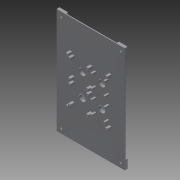
# Autodesk Inventor part: SimpleLensPlane
Saved by Autodesk Inventor 2015 (Build 190159000, 159)
## iProperties
Created: 2015-03-20
Part Number: SimpleLensPlane
Material: NylonD2W
Document SubType Name: Modeling
Designer: Akovo_000
Density: 0.93 g/cm^3
Appearance: Nylon 6
Mass: 35.1863 g
Surface Area: 486.293 cm^2
Volume: 37.8348 cm^3
Author: Akovo_000
Autodesk Inventor part; units mm, degrees
ref_plane "YZ Plane" through (0, 0, 0) normal (1, 0, 0) x (0, 1, 0)
ref_plane "XZ Plane" through (0, 0, 0) normal (0, 1, 0) x (-1, 0, 0)
ref_plane "Main Work Pane" through (0, 2.75, 7) normal (0, 1, 0) x (-1, 0, 0)
sketch "Panel" plane through (0, 2.75, 7) normal (0, 1, 0) x (-1, 0, 0)
  circle A0 centre (9.841, 27.1334) radius 5.8
  circle A1 centre (9.841, -11.8666) radius 5.8
  circle A2 centre (43.641, -11.8666) radius 5.8
  circle A3 centre (43.641, 27.1334) radius 5.8
  line L0 (61.641, 45.1334) -> (25.641, 45.1334)
  line L1 (25.641, 45.1334) -> (25.641, 9.1334)
  line L2 (25.641, 9.1334) -> (61.641, 9.1334)
  line L3 (61.641, 9.1334) -> (61.641, 45.1334)
  line L4 (61.641, 45.1334) -> (25.641, 9.1334) construction
  line L5 (25.641, 45.1334) -> (61.641, 9.1334) construction
  line L6 (61.641, 6.1334) -> (25.641, 6.1334)
  line L7 (25.641, 6.1334) -> (25.641, -29.8666)
  line L8 (25.641, -29.8666) -> (61.641, -29.8666)
  line L9 (61.641, -29.8666) -> (61.641, 6.1334)
  line L10 (61.641, 6.1334) -> (25.641, -29.8666) construction
  line L11 (25.641, 6.1334) -> (61.641, -29.8666) construction
  line L12 (22.641, 39.9334) -> (-2.959, 39.9334)
  line L13 (-2.959, 39.9334) -> (-2.959, 14.3334)
  line L14 (-2.959, 14.3334) -> (22.641, 14.3334)
  line L15 (22.641, 14.3334) -> (22.641, 39.9334)
  line L16 (22.641, 39.9334) -> (-2.959, 14.3334) construction
  line L17 (-2.959, 39.9334) -> (22.641, 14.3334) construction
  line L18 (22.641, 0.9334) -> (-2.959, 0.9334)
  line L19 (-2.959, 0.9334) -> (-2.959, -24.6666)
  line L20 (-2.959, -24.6666) -> (22.641, -24.6666)
  line L21 (22.641, -24.6666) -> (22.641, 0.9334)
  line L22 (22.641, 0.9334) -> (-2.959, -24.6666) construction
  line L23 (-2.959, 0.9334) -> (22.641, -24.6666) construction
  line L24 (61.641, -29.8666) -> (61.641, 45.1334)
  line L25 (61.641, 45.1334) -> (-2.959, 45.1334)
  line L26 (-2.959, 45.1334) -> (-2.959, -29.8666)
  line L27 (-2.959, -29.8666) -> (61.641, -29.8666)
  line L28 (88.341, -83.8666) -> (-29.659, -83.8666)
  line L29 (-29.659, -83.8666) -> (-29.659, 99.1334)
  line L30 (-29.659, 99.1334) -> (88.341, 99.1334)
  line L31 (88.341, 99.1334) -> (88.341, -83.8666)
  line L32 (43.641, 21.3334) -> (43.641, -6.0666) construction
  line L33 (37.841, 27.1334) -> (15.641, 27.1334) construction
  line L34 (9.841, 21.3334) -> (9.841, -6.0666) construction
  line L35 (15.641, -11.8666) -> (37.841, -11.8666) construction
  line L36 (17.4252, 99.1334) -> (17.4252, 45.1334) construction
  line L37 (17.4252, -29.8666) -> (17.4252, -83.8666) construction
  line L38 (61.641, 7.6334) -> (88.341, 7.6334) construction
  line L39 (-2.959, 7.6334) -> (-29.659, 7.6334) construction
  circle A4 centre (80.841, 91.1334) radius 2
  circle A5 centre (-22.159, 91.1334) radius 2
  circle A6 centre (80.841, -75.8666) radius 2
  circle A7 centre (-22.159, -75.8666) radius 2
  line L40 (67.962, 75.8227) -> (67.962, -63.4589)
  line L41 (67.962, -63.4589) -> (-9.8153, -63.4589)
  line L42 (-9.8153, -63.4589) -> (-9.8153, 75.8227)
  line L43 (-9.8153, 75.8227) -> (67.962, 75.8227)
  line L44 (-22.159, 99.1334) -> (-22.159, 91.1334) construction
  line L45 (-22.159, 91.1334) -> (-29.659, 91.1334) construction
  line L46 (80.841, 99.1334) -> (80.841, 91.1334) construction
  line L47 (80.841, 91.1334) -> (88.341, 91.1334) construction
  line L48 (88.341, -75.8666) -> (80.841, -75.8666) construction
  line L49 (80.841, -75.8666) -> (80.841, -83.8666) construction
  line L50 (-22.159, -83.8666) -> (-22.159, -75.8666) construction
  line L51 (-22.159, -75.8666) -> (-29.659, -75.8666) construction
  dimension "d337" = 11.6
  dimension "d490" = 36
  dimension "d491" = 36
  dimension "d494" = 3
  dimension "d495" = 25.6
  dimension "d496" = 25.6
  dimension "d497" = 3
  dimension "d498" = 0
  dimension "d593" = 4
  dimension "d674" = 183
  dimension "d675" = 118
  dimension "d676" = 7.5
  dimension "d677" = 8
  constraints: 104 end point, 20 perpendicular, 14 equal length, 12 midpoint, 12 parallel, 12 point on line, 8 centre point, 8 point on circle, 6 equal radius, 6 line through centre, 5 horizontal, 3 vertical, 2 collinear, 3 other
  measures "d337" diameter of A2
  measures "d490" distance of L2.end L1.end
  measures "d491" distance of L1.end L0.end
  measures "d494" distance between parallel lines of L6 L2
  measures "d495" distance of L14.end L13.end
  measures "d496" distance of L13.end L12.end
  measures "d497" distance between parallel lines of L21 L7
  measures "d498" distance between parallel lines of L26 L13
  measures "d593" diameter of A4
  measures "d674" distance between parallel lines of L28 L30
  measures "d675" distance between parallel lines of L29 L31
  measures "d676" distance of L44.end L45.end
  measures "d677" distance of L44.start L44.end
extrude "FlatPlane" add sketch "Panel" along normal blind 1.5 contours L3 L2 L1 L0 | L1 L2 L24 L6 L7 L27 L26 L20 L21 L18 L14 L15 L12 L25 | L9 L8 L7 L6 | L12 L15 L14 L13 | L18 L21 L20 L19 | L28 L29 L30 L31 | L40 L41 L42 L43
sketch "BoardSuport" plane through (0, 2.75, 7) normal (0, -1, 0) x (1, 0, 0)
  line L0 (-59.141, 42.6334) -> (-28.141, 42.6334) construction
  line L1 (-28.141, 42.6334) -> (-28.141, 11.6334) construction
  line L2 (-28.141, 11.6334) -> (-59.141, 11.6334) construction
  line L3 (-59.141, 11.6334) -> (-59.141, 42.6334) construction
  circle A0 centre (-43.641, 27.1334) radius 5.8
  line L4 (-59.141, 42.6334) -> (-28.141, 11.6334) construction
  line L5 (-28.141, 42.6334) -> (-59.141, 11.6334) construction
  line L6 (-59.141, 3.6334) -> (-28.141, 3.6334) construction
  line L7 (-28.141, 3.6334) -> (-28.141, -27.3666) construction
  line L8 (-28.141, -27.3666) -> (-59.141, -27.3666) construction
  line L9 (-59.141, -27.3666) -> (-59.141, 3.6334) construction
  circle A1 centre (-43.641, -11.8666) radius 5.8
  line L10 (-59.141, 3.6334) -> (-28.141, -27.3666) construction
  line L11 (-28.141, 3.6334) -> (-59.141, -27.3666) construction
  line L12 (-21.091, 38.3834) -> (1.409, 38.3834) construction
  line L13 (1.409, 38.3834) -> (1.409, 15.8834) construction
  line L14 (1.409, 15.8834) -> (-21.091, 15.8834) construction
  line L15 (-21.091, 15.8834) -> (-21.091, 38.3834) construction
  circle A2 centre (-9.841, 27.1334) radius 5.8
  line L16 (-21.091, 38.3834) -> (1.409, 15.8834) construction
  line L17 (1.409, 38.3834) -> (-21.091, 15.8834) construction
  line L18 (-21.091, -0.6166) -> (1.409, -0.6166) construction
  line L19 (1.409, -0.6166) -> (1.409, -23.1166) construction
  line L20 (1.409, -23.1166) -> (-21.091, -23.1166) construction
  line L21 (-21.091, -23.1166) -> (-21.091, -0.6166) construction
  circle A3 centre (-9.841, -11.8666) radius 5.8
  line L22 (-21.091, -0.6166) -> (1.409, -23.1166) construction
  line L23 (1.409, -0.6166) -> (-21.091, -23.1166) construction
  line L24 (-61.241, 5.7334) -> (-57.041, 5.7334)
  line L25 (-57.041, 5.7334) -> (-57.041, 1.5334)
  line L26 (-57.041, 1.5334) -> (-61.241, 1.5334)
  line L27 (-61.241, 1.5334) -> (-61.241, 5.7334)
  line L28 (-61.241, 5.7334) -> (-57.041, 1.5334) construction
  line L29 (-57.041, 5.7334) -> (-61.241, 1.5334) construction
  line L30 (-61.241, 13.7334) -> (-57.041, 13.7334)
  line L31 (-57.041, 13.7334) -> (-57.041, 9.5334)
  line L32 (-57.041, 9.5334) -> (-61.241, 9.5334)
  line L33 (-61.241, 9.5334) -> (-61.241, 13.7334)
  line L34 (-61.241, 13.7334) -> (-57.041, 9.5334) construction
  line L35 (-57.041, 13.7334) -> (-61.241, 9.5334) construction
  line L36 (-30.241, 13.7334) -> (-26.041, 13.7334)
  line L37 (-26.041, 13.7334) -> (-26.041, 9.5334)
  line L38 (-26.041, 9.5334) -> (-30.241, 9.5334)
  line L39 (-30.241, 9.5334) -> (-30.241, 13.7334)
  line L40 (-30.241, 13.7334) -> (-26.041, 9.5334) construction
  line L41 (-26.041, 13.7334) -> (-30.241, 9.5334) construction
  line L42 (-30.241, 44.7334) -> (-26.041, 44.7334)
  line L43 (-26.041, 44.7334) -> (-26.041, 40.5334)
  line L44 (-26.041, 40.5334) -> (-30.241, 40.5334)
  line L45 (-30.241, 40.5334) -> (-30.241, 44.7334)
  line L46 (-30.241, 44.7334) -> (-26.041, 40.5334) construction
  line L47 (-26.041, 44.7334) -> (-30.241, 40.5334) construction
  line L48 (-61.241, 44.7334) -> (-57.041, 44.7334)
  line L49 (-57.041, 44.7334) -> (-57.041, 40.5334)
  line L50 (-57.041, 40.5334) -> (-61.241, 40.5334)
  line L51 (-61.241, 40.5334) -> (-61.241, 44.7334)
  line L52 (-61.241, 44.7334) -> (-57.041, 40.5334) construction
  line L53 (-57.041, 44.7334) -> (-61.241, 40.5334) construction
  line L54 (-30.241, 5.7334) -> (-26.041, 5.7334)
  line L55 (-26.041, 5.7334) -> (-26.041, 1.5334)
  line L56 (-26.041, 1.5334) -> (-30.241, 1.5334)
  line L57 (-30.241, 1.5334) -> (-30.241, 5.7334)
  line L58 (-30.241, 5.7334) -> (-26.041, 1.5334) construction
  line L59 (-26.041, 5.7334) -> (-30.241, 1.5334) construction
  line L60 (-30.241, -25.2666) -> (-26.041, -25.2666)
  line L61 (-26.041, -25.2666) -> (-26.041, -29.4666)
  line L62 (-26.041, -29.4666) -> (-30.241, -29.4666)
  line L63 (-30.241, -29.4666) -> (-30.241, -25.2666)
  line L64 (-30.241, -25.2666) -> (-26.041, -29.4666) construction
  line L65 (-26.041, -25.2666) -> (-30.241, -29.4666) construction
  line L66 (-61.241, -25.2666) -> (-57.041, -25.2666)
  line L67 (-57.041, -25.2666) -> (-57.041, -29.4666)
  line L68 (-57.041, -29.4666) -> (-61.241, -29.4666)
  line L69 (-61.241, -29.4666) -> (-61.241, -25.2666)
  line L70 (-61.241, -25.2666) -> (-57.041, -29.4666) construction
  line L71 (-57.041, -25.2666) -> (-61.241, -29.4666) construction
  line L72 (-22.591, -21.6166) -> (-19.591, -21.6166)
  line L73 (-19.591, -21.6166) -> (-19.591, -24.6166)
  line L74 (-19.591, -24.6166) -> (-22.591, -24.6166)
  line L75 (-22.591, -24.6166) -> (-22.591, -21.6166)
  line L76 (-22.591, -21.6166) -> (-19.591, -24.6166) construction
  line L77 (-19.591, -21.6166) -> (-22.591, -24.6166) construction
  line L78 (-0.091, -21.6166) -> (2.909, -21.6166)
  line L79 (2.909, -21.6166) -> (2.909, -24.6166)
  line L80 (2.909, -24.6166) -> (-0.091, -24.6166)
  line L81 (-0.091, -24.6166) -> (-0.091, -21.6166)
  line L82 (-0.091, -21.6166) -> (2.909, -24.6166) construction
  line L83 (2.909, -21.6166) -> (-0.091, -24.6166) construction
  line L84 (-0.091, 0.8834) -> (2.909, 0.8834)
  line L85 (2.909, 0.8834) -> (2.909, -2.1166)
  line L86 (2.909, -2.1166) -> (-0.091, -2.1166)
  line L87 (-0.091, -2.1166) -> (-0.091, 0.8834)
  line L88 (-0.091, 0.8834) -> (2.909, -2.1166) construction
  line L89 (2.909, 0.8834) -> (-0.091, -2.1166) construction
  line L90 (-22.591, 0.8834) -> (-19.591, 0.8834)
  line L91 (-19.591, 0.8834) -> (-19.591, -2.1166)
  line L92 (-19.591, -2.1166) -> (-22.591, -2.1166)
  line L93 (-22.591, -2.1166) -> (-22.591, 0.8834)
  line L94 (-22.591, 0.8834) -> (-19.591, -2.1166) construction
  line L95 (-19.591, 0.8834) -> (-22.591, -2.1166) construction
  line L96 (-22.591, 14.3834) -> (-19.591, 14.3834)
  line L97 (-19.591, 14.3834) -> (-19.591, 17.3834)
  line L98 (-19.591, 17.3834) -> (-22.591, 17.3834)
  line L99 (-22.591, 17.3834) -> (-22.591, 14.3834)
  line L100 (-22.591, 14.3834) -> (-19.591, 17.3834) construction
  line L101 (-19.591, 14.3834) -> (-22.591, 17.3834) construction
  line L102 (2.909, 14.3834) -> (-0.091, 14.3834)
  line L103 (-0.091, 14.3834) -> (-0.091, 17.3834)
  line L104 (-0.091, 17.3834) -> (2.909, 17.3834)
  line L105 (2.909, 17.3834) -> (2.909, 14.3834)
  line L106 (2.909, 14.3834) -> (-0.091, 17.3834) construction
  line L107 (-0.091, 14.3834) -> (2.909, 17.3834) construction
  line L108 (2.909, 39.8834) -> (-0.091, 39.8834)
  line L109 (-0.091, 39.8834) -> (-0.091, 36.8834)
  line L110 (-0.091, 36.8834) -> (2.909, 36.8834)
  line L111 (2.909, 36.8834) -> (2.909, 39.8834)
  line L112 (2.909, 39.8834) -> (-0.091, 36.8834) construction
  line L113 (-0.091, 39.8834) -> (2.909, 36.8834) construction
  line L114 (-22.591, 39.8834) -> (-19.591, 39.8834)
  line L115 (-19.591, 39.8834) -> (-19.591, 36.8834)
  line L116 (-19.591, 36.8834) -> (-22.591, 36.8834)
  line L117 (-22.591, 36.8834) -> (-22.591, 39.8834)
  line L118 (-22.591, 39.8834) -> (-19.591, 36.8834) construction
  line L119 (-19.591, 39.8834) -> (-22.591, 36.8834) construction
  arc A4 (-59.141, 40.5334) -> (-57.041, 42.6334) centre (-59.141, 42.6334) ccw
  arc A5 (-30.241, 42.6334) -> (-28.141, 40.5334) centre (-28.141, 42.6334) ccw
  arc A6 (-28.141, 13.7334) -> (-30.241, 11.6334) centre (-28.141, 11.6334) ccw
  arc A7 (-57.041, 11.6334) -> (-59.141, 13.7334) centre (-59.141, 11.6334) ccw
  arc A8 (-59.141, 1.5334) -> (-57.041, 3.6334) centre (-59.141, 3.6334) ccw
  arc A9 (-57.041, -27.3666) -> (-59.141, -25.2666) centre (-59.141, -27.3666) ccw
  arc A10 (-28.141, -25.2666) -> (-30.241, -27.3666) centre (-28.141, -27.3666) ccw
  arc A11 (-19.591, -23.1166) -> (-21.091, -21.6166) centre (-21.091, -23.1166) ccw
  arc A12 (1.409, -21.6166) -> (-0.091, -23.1166) centre (1.409, -23.1166) ccw
  arc A13 (-0.091, -0.6166) -> (1.409, -2.1166) centre (1.409, -0.6166) ccw
  arc A14 (-21.091, -2.1166) -> (-19.591, -0.6166) centre (-21.091, -0.6166) ccw
  arc A15 (-30.241, 3.6334) -> (-28.141, 1.5334) centre (-28.141, 3.6334) ccw
  arc A16 (-21.091, 36.8834) -> (-19.591, 38.3834) centre (-21.091, 38.3834) ccw
  arc A17 (-19.591, 15.8834) -> (-21.091, 17.3834) centre (-21.091, 15.8834) ccw
  arc A18 (1.409, 17.3834) -> (-0.091, 15.8834) centre (1.409, 15.8834) ccw
  arc A19 (-0.091, 38.3834) -> (1.409, 36.8834) centre (1.409, 38.3834) ccw
  circle A20 centre (-59.141, 42.6334) radius 0.9
  circle A21 centre (-59.141, 11.6334) radius 0.9
  circle A22 centre (-28.141, 11.6334) radius 0.9
  circle A23 centre (-28.141, 42.6334) radius 0.9
  circle A24 centre (-59.141, 3.6334) radius 0.9
  circle A25 centre (-59.141, -27.3666) radius 0.9
  circle A26 centre (-28.141, -27.3666) radius 0.9
  circle A27 centre (-28.141, 3.6334) radius 0.9
  circle A28 centre (-21.091, -0.6166) radius 0.9
  circle A29 centre (-21.091, -23.1166) radius 0.9
  circle A30 centre (1.409, -23.1166) radius 0.9
  circle A31 centre (1.409, -0.6166) radius 0.9
  circle A32 centre (1.409, 15.8834) radius 0.9
  circle A33 centre (-21.091, 15.8834) radius 0.9
  circle A34 centre (1.409, 38.3834) radius 0.9
  circle A35 centre (-21.091, 38.3834) radius 0.9
  circle A36 centre (-43.641, 27.1334) radius 5.8 projected
  circle A37 centre (-9.841, 27.1334) radius 5.8 projected
  circle A38 centre (-43.641, -11.8666) radius 5.8 projected
  circle A39 centre (-9.841, -11.8666) radius 5.8 projected
  line L120 (-61.241, 44.7334) -> (2.909, 44.7334) construction
  line L121 (2.909, 44.7334) -> (2.909, -29.4666) construction
  line L122 (2.909, -29.4666) -> (-61.241, -29.4666) construction
  line L123 (-61.241, -29.4666) -> (-61.241, 44.7334) construction
  line L124 (-61.241, 44.7334) -> (-65.241, 44.7334)
  line L125 (-65.241, 44.7334) -> (-65.241, 48.7334)
  line L126 (-65.241, 48.7334) -> (-61.241, 48.7334)
  line L127 (-61.241, 48.7334) -> (-61.241, 44.7334)
  line L128 (-61.241, -29.4666) -> (-65.241, -29.4666)
  line L129 (-65.241, -29.4666) -> (-65.241, -33.4666)
  line L130 (-65.241, -33.4666) -> (-61.241, -33.4666)
  line L131 (-61.241, -33.4666) -> (-61.241, -29.4666)
  line L132 (2.909, -29.4666) -> (6.909, -29.4666)
  line L133 (6.909, -29.4666) -> (6.909, -33.4666)
  line L134 (6.909, -33.4666) -> (2.909, -33.4666)
  line L135 (2.909, -33.4666) -> (2.909, -29.4666)
  line L136 (2.909, 44.7334) -> (6.909, 44.7334)
  line L137 (6.909, 44.7334) -> (6.909, 48.7334)
  line L138 (6.909, 48.7334) -> (2.909, 48.7334)
  line L139 (2.909, 48.7334) -> (2.909, 44.7334)
  circle A40 centre (5.4519, 46.9805) radius 0.9
  circle A41 centre (-62.6981, 46.9805) radius 0.9
  circle A42 centre (-62.6981, -31.2195) radius 0.9
  circle A43 centre (5.4519, -31.2195) radius 0.9
  dimension "d543" = 22.5
  dimension "d545" = 4.2
  dimension "d546" = 3
  dimension "d547" = 1.8
  dimension "d548" = 1.8
  dimension "d642" = 31
  dimension "d643" = 31
  dimension "d644" = 22.5
  dimension "d645" = 0
  dimension "d646" = 0
  dimension "d647" = 11.6
  dimension "d662" = 4
  dimension "d665" = 72.15
  dimension "d666" = 82.2
  dimension "d667" = 1.8
  constraints: 280 end point, 76 midpoint, 50 parallel, 40 centre point, 32 point on circle, 25 horizontal, 25 perpendicular, 21 equal length, 20 equal radius, 20 point on line, 16 tangent, 15 coincident, 3 concentric
  measures "d543" distance of L12.end L13.end
  measures "d545" distance between parallel lines of L24 L26
  measures "d546" distance between parallel lines of L80 L78
  measures "d547" diameter of A25
  measures "d548" diameter of A30
  measures "d642" distance of L0.end L0.start
  measures "d643" distance of L2.end L0.start
  measures "d644" distance of L12.start L12.end
  measures "d645" distance of A0.centre A36.centre
  measures "d646" distance of A36.centre A0.centre
  measures "d647" diameter of A0
  measures "d662" distance of L125.end L126.end
  measures "d665" distance between parallel lines of L129 L133
  measures "d666" distance between parallel lines of L138 L134
  measures "d667" diameter of A40
extrude "BoardSupport3D" add sketch "BoardSuport" along normal blind 7.2 contours L24 L25 A8 L26 L27 | L25 L26 A8 | L30 A7 L31 L32 L33 | L30 L31 A7 | L36 A6 L39 | L36 L37 L38 L39 A6 | L42 L43 L44 A5 L45 | A5 L44 L45 | L48 L49 A4 L50 L51 | L124 L125 L126 L127 | L49 L50 A4 | L54 L55 L56 A15 L57 | A15 L56 L57 | L60 A10 L63 | L60 L61 L62 L63 A10 | L131 L130 L129 L128 | L66 A9 L67 L68 L69 | L66 L67 A9 | L72 A11 L73 L74 L75 | L72 L73 A11 | L78 A12 L81 | L78 L79 L80 L81 A12 | L84 L85 L86 A13 L87 | A13 L86 L87 | L90 L91 A14 L92 L93 | L91 L92 A14 | L99 L98 A17 L97 L96 | A17 L98 L97 | L102 L103 A18 L104 L105 | L103 L104 A18 | L111 L110 A19 L109 L108 | A19 L110 L109 | L114 L115 A16 L116 L117 | L115 L116 A16 | L132 L133 L134 L135 | L139 L138 L137 L136
sketch "Lens and screwcover" plane through (0, 4.25, 7) normal (0, 1, 0) x (1, 0, 0)
  circle A0 centre (-43.641, -27.1334) radius 5.8
  circle A1 centre (-43.641, -27.1334) radius 5.8
  circle A2 centre (-9.841, -27.1334) radius 5.8
  circle A3 centre (-9.841, -27.1334) radius 5.8
  circle A4 centre (-9.841, 11.8666) radius 5.8
  circle A5 centre (-9.841, 11.8666) radius 5.8
  circle A6 centre (-43.641, 11.8666) radius 5.8
  circle A7 centre (-43.641, 11.8666) radius 5.8
  circle A8 centre (-43.641, -27.1334) radius 8.3
  circle A9 centre (-9.841, -27.1334) radius 8.3
  circle A10 centre (-9.841, 11.8666) radius 8.3
  circle A11 centre (-43.641, 11.8666) radius 8.3
  line L0 (29.659, 83.8666) -> (14.659, 83.8666)
  line L1 (14.659, 83.8666) -> (14.659, 68.8666)
  line L2 (14.659, 68.8666) -> (29.659, 68.8666)
  line L3 (29.659, 68.8666) -> (29.659, 83.8666)
  line L4 (-88.341, 83.8666) -> (-73.341, 83.8666)
  line L5 (-73.341, 83.8666) -> (-73.341, 68.8666)
  line L6 (-73.341, 68.8666) -> (-88.341, 68.8666)
  line L7 (-88.341, 68.8666) -> (-88.341, 83.8666)
  line L8 (-88.341, -99.1334) -> (-73.341, -99.1334)
  line L9 (-73.341, -99.1334) -> (-73.341, -84.1334)
  line L10 (-73.341, -84.1334) -> (-88.341, -84.1334)
  line L11 (-88.341, -84.1334) -> (-88.341, -99.1334)
  line L12 (29.659, -99.1334) -> (14.659, -99.1334)
  line L13 (14.659, -99.1334) -> (14.659, -84.1334)
  line L14 (14.659, -84.1334) -> (29.659, -84.1334)
  line L15 (29.659, -84.1334) -> (29.659, -99.1334)
  circle A12 centre (-43.641, -27.1334) radius 5.8 projected
  circle A13 centre (-43.641, 11.8666) radius 5.8 projected
  circle A14 centre (-9.841, 11.8666) radius 5.8 projected
  circle A15 centre (-9.841, -27.1334) radius 5.8 projected
  circle A16 centre (-80.841, 75.8666) radius 2 projected
  circle A17 centre (-80.841, 75.8666) radius 2
  circle A18 centre (22.159, 75.8666) radius 2 projected
  circle A19 centre (22.159, 75.8666) radius 2
  circle A20 centre (22.159, -91.1334) radius 2 projected
  circle A21 centre (22.159, -91.1334) radius 2
  circle A22 centre (-80.841, -91.1334) radius 2 projected
  circle A23 centre (-80.841, -91.1334) radius 2
  point P0 (0, 7)
  dimension "d551" = 2.5
  dimension "d600" = 15
  dimension "d601" = 15
  constraints: 32 end point, 16 centre point, 12 coincident, 8 parallel, 6 equal length, 4 concentric, 4 horizontal, 4 perpendicular, 3 equal radius, 2 point on line
  measures "d551" radial gap between concentric circles of A8 A0
  measures "d600" distance of L2.end L1.end
  measures "d601" distance of L1.end L0.end
extrude "Extrusion15" add sketch "Lens and screwcover" along normal blind 3.5
body "Solid3"
